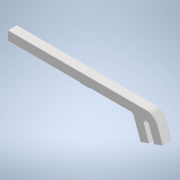
# Autodesk Inventor part: grip_N_fix
Saved by Autodesk Inventor 2021 (Build 250183000, 183)
## iProperties
Created: 2021-05-09
Part Number: grip_N_fix
Material: Generic
Document SubType Name: Modeling
Designer: Alsayaary
Density: 1 g/cm^3
Appearance: Default
Author: Abdulrahman
Autodesk Inventor part; units mm, degrees
ref_plane "YZ Plane" through (0, 0, 0) normal (1, 0, 0) x (0, 1, 0)
ref_plane "XZ Plane" through (0, 0, 0) normal (0, 1, 0) x (-1, 0, 0)
ref_plane "XY Plane" through (0, 0, 0) normal (0, 0, 1) x (1, 0, 0)
sketch "Sketch1" plane through (0, 0, 0) normal (0, 0, 1) x (1, 0, 0)
  line L0 (107.3767, 69.0782) -> (130.453, 5.6766)
  line L1 (130.453, 5.6766) -> (158.6438, 15.9372)
  line L2 (158.6438, 15.9372) -> (141.5428, 62.9218)
  arc A0 (158.4572, 69.0782) -> (141.5428, 62.9218) centre (150, 66) ccw
  line L3 (158.4572, 69.0782) -> (175.5582, 22.0936)
  line L4 (175.5582, 22.0936) -> (203.749, 32.3542)
  line L5 (203.749, 32.3542) -> (186.648, 79.3388)
  arc A1 (186.648, 79.3388) -> (150, 105) centre (150, 66) ccw
  line L6 (98.9195, 75) -> (-201.0805, 75)
  line L7 (150, 105) -> (-201.0805, 105)
  line L8 (-201.0805, 105) -> (-201.0805, 75)
  line L9 (0, 131.7977) -> (0, -15.3436) projected
  line L10 (-282.0464, 0) -> (284.7149, 0) projected
  arc A2 (107.3767, 69.0782) -> (98.9195, 75) centre (98.9195, 66) ccw
  dimension "d38" = 30
  dimension "d39" = 30
  dimension "d40" = 9
  dimension "d47" = 30
  dimension "d53" = 9
  dimension "d56" = 300
  dimension "d58" = 150
  dimension "d59" = 50
  dimension "d60" = 20
  dimension "d61" = 75
  constraints: 18 end point, 6 perpendicular, 6 point on circle, 6 tangent, 3 centre point, 1 coincident, 1 collinear, 1 parallel
  measures "d38" distance of L3.end L4.end
  measures "d39" distance of L0.end L1.end
  measures "d40" radius of A0
  measures "d47" distance of L7.end L6.end
  measures "d53" radius of A2
  measures "d56" distance of L6.start L6.end
  measures "d58" distance from line of L9 A0.centre
  measures "d59" distance from line of A0.centre L4
  measures "d60" angle of L1 L6
  measures "d61" distance between parallel lines of L10 L6
extrude "Extrusion1" add sketch "Sketch1" along normal mid plane 30
sketch "Sketch4" plane through (0, 0, 0) normal (0, 0, 1) x (1, 0, 0)
  line L0 (-201.0805, 75) -> (98.9195, 75) projected
  line L1 (-15, 75) -> (15, 75)
  line L2 (-15, 75) -> (-15, 74)
  line L3 (-15, 74) -> (15, 74)
  line L4 (15, 74) -> (15, 75)
  line L5 (0, 90) -> (0, -15) projected
  point P0 (0, 0)
  dimension "d62" = 30
  dimension "d63" = 15
  dimension "d64" = 1
  constraints: 8 end point, 2 perpendicular, 2 point on line, 1 vertical
  measures "d62" distance of L2.end L3.end
  measures "d63" distance between parallel lines of L5 L2
  measures "d64" distance of L3.end L1.end
extrude "Extrusion4" add sketch "Sketch4" along normal mid plane 30
fillet "Fillet1" radius 2 14 edges at (-108.0403, 75, 15) (104.0817, 73.3724, 15) (118.9148, 37.3774, 15) (56.9597, 75, 15) (-108.0403, 75, -15) (104.0817, 73.3724, -15) (118.9148, 37.3774, -15) (56.9597, 75, -15) (172.3695, 97.9469, -15) (195.1985, 55.8465, -15) (-25.5403, 105, -15) (172.3695, 97.9469, 15) (195.1985, 55.8465, 15) (-25.5403, 105, 15)
sketch "Sketch5" plane through (-201.0805, 77, -15) normal (-1, 0, 0) x (0, 0, 1)
  line L0 (27.5, 25.5) -> (2.5, 25.5)
  line L1 (2.5, 25.5) -> (2.5, 0.5)
  line L2 (2.5, 0.5) -> (27.5, 0.5)
  line L3 (27.5, 0.5) -> (27.5, 25.5)
  line L4 (2, 28) -> (28, 28) projected
  line L5 (0, 0) -> (0, 26) projected
  line L6 (2, -2) -> (28, -2) projected
  line L7 (30, 26) -> (30, 0) projected
  point P0 (15, -77)
  dimension "d68" = 2.5
  dimension "d69" = 2.5
  dimension "d70" = 2.5
  dimension "d71" = 2.5
  constraints: 8 end point, 2 parallel, 1 horizontal, 1 perpendicular
  measures "d68" distance between parallel lines of L0 L4
  measures "d69" distance between parallel lines of L5 L1
  measures "d70" distance between parallel lines of L6 L2
  measures "d71" distance between parallel lines of L7 L3
extrude "Extrusion5" cut sketch "Sketch5" against normal blind 400
fillet "Fillet2" radius 2 4 edges at (-6.8816, 77.5, 12.5) (-6.8816, 77.5, -12.5) (-18.671, 102.5, -12.5) (-18.671, 102.5, 12.5)
equation "\"d39\" = d38"
equation "\"secure_arm_radii\" = 9"
equation "\"rack_tooth_thickness\" = 5"
equation "\"rack_tooth_addendum\" = 5"
equation "\"rack_tooth_dedendum\" = 5"
equation "\"hoop_bearing_length\" = 5deg"
equation "\"secure_arm_angle\" = 20deg"
equation "\"hoop_tabs_thickness\" = 6"
equation "\"hoop_tabs_hole\" = 12"
equation "\"support_baseClamp_thickness\" = 8"
equation "\"support_frame_endHoleBuffer\" = 25"
equation "\"support_frame_squareBarThickness\" = 5"
equation "\"support_baseClamp_sleeveSweepTerminationAngle\" = 55deg"
equation "\"support_baseClamp_sleeveHoleDiameter\" = 12"
equation "\"support_frame_squareBarFillet\" = 2"
equation "\"support_baseClamp_platformWidthBuffer\" = 0"
equation "\"support_baseClamp_platformThickness\" = 15"
equation "\"support_baseClamp_platformLengthBuffer\" = 35"
equation "\"hoop_angle_z\" = 45deg"
equation "\"hoop_cable_diam\" = 5"
equation "\"hoop_cable_pulley_diam\" = 22"
equation "\"wheelchair_deployed_width\" = 635"
equation "\"wheelchair_deployed_height\" = 914"
equation "\"wheelchair_deployed_length\" = 1067"
equation "\"sm_varx_pinPlate_thickness\" = 5"
equation "\"sm_varx_member_tolerance\" = 0.5"
equation "\"sm_varx_pinPlate_holeDiameter\" = 5"
equation "\"sm_varx_squareBarThickness\" = 2.5"
body "Solid1"
